Autodesk Fusion 360 part; units mm, degrees
(part 8 of 8)
  spline S1829 degree 3 poles (-135.1816, -10.4199) (-135.1816, -9.9969) (-135.975, -9.9438) (-136.5053, -8.9646) knots -1 -1 -1 -1 0 0 0 0
  line L415 (-136.5053, -8.9646) -> (-141.2417, 0.3483)
  spline S1830 degree 3 poles (44.6732, -11.214) (42.5035, -11.214) (42.0799, -11.2933) (39.5925, -11.2933) knots 0 0 0 0 1 1 1 1
  spline S1831 degree 3 poles (39.5925, -11.2933) (42.0799, -11.2933) (42.5035, -11.214) (44.6732, -11.214) knots -1 -1 -1 -1 0 0 0 0
  spline S1832 degree 3 poles (30.6505, -5.2874) (30.6505, -1.5566) (34.0109, 0.7979) (39.3034, 0.7979) knots 0 0 0 0 1 1 1 1
  spline S1833 degree 3 poles (39.3034, 0.7979) (34.0109, 0.7979) (30.6505, -1.5566) (30.6505, -5.2874) knots -1 -1 -1 -1 0 0 0 0
  spline S1834 degree 3 poles (48.6433, 5.6399) (48.6433, 5.2166) (47.2121, 5.2959) (47.2121, 4.1847) knots 0 0 0 0 1 1 1 1
  spline S1835 degree 3 poles (47.2121, 4.1847) (47.2121, 5.2959) (48.6433, 5.2166) (48.6433, 5.6399) knots -1 -1 -1 -1 0 0 0 0
  spline S1836 degree 3 poles (-148.0434, 5.6402) (-148.0434, 5.9575) (-147.7524, 6.5133) (-147.5411, 6.5133) knots 0 0 0 0 1 1 1 1
  spline S1837 degree 3 poles (-147.5411, 6.5133) (-147.7524, 6.5133) (-148.0434, 5.9575) (-148.0434, 5.6402) knots -1 -1 -1 -1 0 0 0 0
  spline S1838 degree 3 poles (-136.5053, -8.9646) (-135.975, -9.9438) (-135.1816, -9.9969) (-135.1816, -10.4199) knots 0 0 0 0 1 1 1 1
  spline S1839 degree 3 poles (-135.1816, -10.4199) (-135.1816, -9.9969) (-135.975, -9.9438) (-136.5053, -8.9646) knots -1 -1 -1 -1 0 0 0 0
  spline S1840 degree 3 poles (-147.5411, 6.5133) (-146.5084, 6.4603) (-145.2127, 6.434) (-143.917, 6.434) knots 0 0 0 0 1 1 1 1
  spline S1841 degree 3 poles (-143.917, 6.434) (-145.2127, 6.434) (-146.5084, 6.4603) (-147.5411, 6.5133) knots -1 -1 -1 -1 0 0 0 0
  spline S1842 degree 3 poles (-135.1816, -10.4199) (-135.1816, -10.7376) (-135.4727, -11.293) (-135.684, -11.293) knots 0 0 0 0 1 1 1 1
  spline S1843 degree 3 poles (-135.684, -11.293) (-135.4727, -11.293) (-135.1816, -10.7376) (-135.1816, -10.4199) knots -1 -1 -1 -1 0 0 0 0
  spline S1844 degree 3 poles (-143.917, 6.434) (-142.6212, 6.434) (-141.3494, 6.4603) (-140.2889, 6.5133) knots 0 0 0 0 1 1 1 1
  spline S1845 degree 3 poles (-140.2889, 6.5133) (-141.3494, 6.4603) (-142.6212, 6.434) (-143.917, 6.434) knots -1 -1 -1 -1 0 0 0 0
  spline S1846 degree 3 poles (-135.684, -11.293) (-136.7445, -11.2404) (-138.0681, -11.2137) (-139.3918, -11.2137) knots 0 0 0 0 1 1 1 1
  spline S1847 degree 3 poles (-139.3918, -11.2137) (-138.0681, -11.2137) (-136.7445, -11.2404) (-135.684, -11.293) knots -1 -1 -1 -1 0 0 0 0
  spline S1848 degree 3 poles (-146.5882, 4.1586) (-146.5882, 5.2961) (-148.0434, 5.2168) (-148.0434, 5.6402) knots 0 0 0 0 1 1 1 1
  spline S1849 degree 3 poles (-148.0434, 5.6402) (-148.0434, 5.2168) (-146.5882, 5.2961) (-146.5882, 4.1586) knots -1 -1 -1 -1 0 0 0 0
  spline S1850 degree 3 poles (-139.3918, -11.2137) (-140.7394, -11.2137) (-142.063, -11.2404) (-143.1235, -11.293) knots 0 0 0 0 1 1 1 1
  spline S1851 degree 3 poles (-143.1235, -11.293) (-142.063, -11.2404) (-140.7394, -11.2137) (-139.3918, -11.2137) knots -1 -1 -1 -1 0 0 0 0
  line L416 (-146.5882, 4.1586) -> (-146.5882, 0.3483)
  line L417 (-146.5882, 0.3483) -> (-146.5882, 4.1586)
  spline S1852 degree 3 poles (-143.1235, -11.293) (-143.3348, -11.293) (-143.598, -10.7376) (-143.598, -10.4199) knots 0 0 0 0 1 1 1 1
  spline S1853 degree 3 poles (-143.598, -10.4199) (-143.598, -10.7376) (-143.3348, -11.293) (-143.1235, -11.293) knots -1 -1 -1 -1 0 0 0 0
  line L418 (-146.5882, 0.3483) -> (-151.3246, -8.9383)
  line L419 (-151.3246, -8.9383) -> (-146.5882, 0.3483)
  spline S1854 degree 3 poles (-143.598, -10.4199) (-143.598, -9.9969) (-142.0351, -9.9438) (-142.5653, -8.9383) knots 0 0 0 0 1 1 1 1
  spline S1855 degree 3 poles (-142.5653, -8.9383) (-142.0351, -9.9438) (-143.598, -9.9969) (-143.598, -10.4199) knots -1 -1 -1 -1 0 0 0 0
  spline S1856 degree 3 poles (-152.6482, -10.4199) (-152.6482, -9.9969) (-151.8548, -9.9438) (-151.3246, -8.9383) knots 0 0 0 0 1 1 1 1
  spline S1857 degree 3 poles (-151.3246, -8.9383) (-151.8548, -9.9438) (-152.6482, -9.9969) (-152.6482, -10.4199) knots -1 -1 -1 -1 0 0 0 0
  line L420 (-145.8506, -2.5091) -> (-142.5653, -8.9383)
  line L421 (-142.5653, -8.9383) -> (-145.8506, -2.5091)
  spline S1858 degree 3 poles (-152.1459, -11.293) (-152.3572, -11.3225) (-152.6482, -10.7376) (-152.6482, -10.4199) knots 0 0 0 0 1 1 1 1
  spline S1859 degree 3 poles (-152.6482, -10.4199) (-152.6482, -10.7376) (-152.3572, -11.3225) (-152.1459, -11.293) knots -1 -1 -1 -1 0 0 0 0
  line L422 (-149.1278, -8.9383) -> (-145.8506, -2.5091)
  line L423 (-145.8506, -2.5091) -> (-149.1278, -8.9383)
  spline S1860 degree 3 poles (-150.3717, -11.2137) (-151.0615, -11.2137) (-151.7472, -11.2404) (-152.1459, -11.293) knots 0 0 0 0 1 1 1 1
  spline S1861 degree 3 poles (-152.1459, -11.293) (-151.7472, -11.2404) (-151.0615, -11.2137) (-150.3717, -11.2137) knots -1 -1 -1 -1 0 0 0 0
  spline S1862 degree 3 poles (-149.1278, -8.9383) (-149.6581, -9.9438) (-148.0992, -9.9969) (-148.0992, -10.4199) knots 0 0 0 0 1 1 1 1
  spline S1863 degree 3 poles (-148.0992, -10.4199) (-148.0992, -9.9969) (-149.6581, -9.9438) (-149.1278, -8.9383) knots -1 -1 -1 -1 0 0 0 0
  spline S1864 degree 3 poles (-148.5736, -11.293) (-148.9962, -11.2404) (-149.686, -11.2137) (-150.3717, -11.2137) knots 0 0 0 0 1 1 1 1
  spline S1865 degree 3 poles (-150.3717, -11.2137) (-149.686, -11.2137) (-148.9962, -11.2404) (-148.5736, -11.293) knots -1 -1 -1 -1 0 0 0 0
  spline S1866 degree 3 poles (-139.8144, 5.6402) (-139.8144, 5.2168) (-141.2417, 5.2961) (-141.2417, 4.1586) knots 0 0 0 0 1 1 1 1
  spline S1867 degree 3 poles (-141.2417, 4.1586) (-141.2417, 5.2961) (-139.8144, 5.2168) (-139.8144, 5.6402) knots -1 -1 -1 -1 0 0 0 0
sketch "Sketch3" plane through (0, 0, 0) normal (0, 0, 1) x (1, 0, 0)
move_body "Move2" bodies 7 20 4 23 21 22 17 10 8 5 16 18 19 6 9 3 to x (1, 0, 0) y (0, 1, 0) z (0, 0, 1) at (-167.0633, -25.6408, 5.9513)
move_body "Move3" bodies 20 21 8 6 18 19 7 5 to x (1, 0, 0) y (0, 1, 0) z (0, 0, 1) at (-155.1525, -24.5373, 4.3298)
